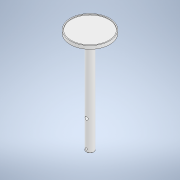
# Autodesk Inventor part: wał_hamulca_dlugi
Saved by Autodesk Inventor 2020 (Build 240168000, 168)
## iProperties
Created: 2020-08-28
Part Number: wał_hamulca_dlugi
Material: ABS Plastic
Document SubType Name: Modeling
Designer: Hesekiel
Density: 1.06 g/cm^3
Appearance: Smooth - White
Mass: 28.992 g
Surface Area: 125.782 cm^2
Volume: 27.351 cm^3
Author: Hesekiel
Autodesk Inventor part; units mm, degrees
ref_plane "YZ Plane" through (0, 0, 0) normal (1, 0, 0) x (0, 1, 0)
ref_plane "XZ Plane" through (0, 0, 0) normal (0, 1, 0) x (-1, 0, 0)
sketch "Sketch1" plane through (0, 0, 0) normal (0, 1, 0) x (-1, 0, 0)
  circle A0 centre (0, 0) radius 5.75
  dimension "d0" = 11.5
  constraints: 1 centre point, 1 coincident
  measures "d0" diameter of A0
extrude "Extrusion1" add sketch "Sketch1" along normal blind 155
sketch "Sketch2" plane through (0, 155, 0) normal (0, 1, 0) x (1, 0, 0)
  circle A0 centre (0, 0) radius 30
  dimension "d3" = 60
  constraints: 1 centre point, 1 coincident
  measures "d3" diameter of A0
extrude "Extrusion2" add sketch "Sketch2" along normal blind 5
sketch "Sketch3" plane through (0, 160, 0) normal (0, 1, 0) x (1, 0, 0)
  circle A0 centre (0, 0) radius 28.6
  dimension "d6" = 57.2
  constraints: 1 centre point, 1 coincident
  measures "d6" diameter of A0
extrude "Extrusion3" cut sketch "Sketch3" against normal blind 1
ref_plane "Work Plane1" through (0, 0, 5.75) normal (0, 0, 1) x (1, 0, 0)
sketch "Sketch4" plane through (0, 0, 5.75) normal (0, 0, 1) x (1, 0, 0)
  line L0 (5.75, 155) -> (-5.75, 155) projected
  line L1 (5.75, 0) -> (-5.75, 0) projected
  line L2 (0, 0) -> (0, 5)
  circle A0 centre (0, 5) radius 1.5
  dimension "d9" = 5
  dimension "d10" = 3
  constraints: 2 end point, 1 centre point, 1 coincident, 1 vertical
  measures "d9" distance of L2.start L2.end
  measures "d10" diameter of A0
extrude "Extrusion4" cut sketch "Sketch4" against normal blind 11.5
chamfer "Chamfer1" distance 1 angle 45 1 edges at (5.75, 0, 0)
sketch "Sketch5" plane through (0, 0, 0) normal (0, 0, 1) x (1, 0, 0)
  line L0 (0, 0) -> (0, 42.5)
  line L1 (0, 42.5) -> (0, 32.5)
  line L2 (0, 42.5) -> (0, 45.5)
  circle A0 centre (0, 45.5) radius 2.5
  dimension "d16" = 42.5
  dimension "d17" = 10
  dimension "d18" = 3
  dimension "d19" = 5
  constraints: 6 end point, 2 point on line, 1 centre point, 1 coincident, 1 vertical
  measures "d16" distance of L0.start L0.end
  measures "d17" distance of L0.end L1.end
  measures "d18" distance of L0.end L2.end
  measures "d19" diameter of A0
extrude "Extrusion5" cut sketch "Sketch5" along normal mid plane 13
body "Solid1"
